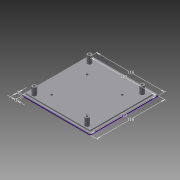
# Autodesk Inventor part: nuccase_top
Saved by Autodesk Inventor 2015 (Build 190159000, 159)
## iProperties
Created: 2016-10-24
Part Number: nuccase_top
Material: Generic
Document SubType Name: Modeling
Designer: Bardo91
Density: 1 g/cm^3
Appearance: Default
Author: Bardo91
Autodesk Inventor part; units mm, degrees
ref_plane "YZ Plane" through (0, 0, 0) normal (1, 0, 0) x (0, 1, 0)
ref_plane "XZ Plane" through (0, 0, 0) normal (0, 1, 0) x (-1, 0, 0)
ref_plane "XY Plane" through (0, 0, 0) normal (0, 0, 1) x (1, 0, 0)
sketch "Sketch1" plane through (0, 0, 0) normal (0, 0, 1) x (1, 0, 0)
  line L0 (0, 0) -> (110, 0)
  line L1 (110, 0) -> (110, 110)
  line L2 (110, 110) -> (0, 110)
  line L3 (0, 110) -> (0, 0)
  line L4 (0, 0) -> (0, -3)
  line L5 (0, -3) -> (-3, -3)
  line L6 (-3, -3) -> (113, -3)
  line L7 (113, -3) -> (113, 113)
  line L8 (113, 113) -> (-3, 113)
  line L9 (-3, 113) -> (-3, -3)
  dimension "d0" = 110
  dimension "d1" = 110
  dimension "d2" = 3
  dimension "d3" = 3
  dimension "d4" = 116
  dimension "d5" = 116
  constraints: 20 end point, 4 parallel, 3 perpendicular, 2 horizontal, 1 vertical
  measures "d0" distance of L2.end L1.end
  measures "d1" distance of L1.end L0.end
  measures "d2" distance of L0.start L4.end
  measures "d3" distance of L4.end L5.end
  measures "d4" distance of L8.end L7.end
  measures "d5" distance of L7.end L6.end
extrude "Extrusion1" add sketch "Sketch1" along normal blind 4 contours L3 L2 L1 L0
extrude "Extrusion2" add sketch "Sketch1" along normal blind 2
sketch "Sketch2" plane through (0, 0, 4) normal (0, 0, 1) x (1, 0, 0)
  line L0 (0, 0) -> (110, 0) projected
  line L1 (55, 0) -> (55, 5)
  line L2 (55, 5) -> (10, 5)
  line L3 (10, 5) -> (100, 5)
  line L4 (100, 5) -> (100, 99)
  line L5 (100, 99) -> (10, 99)
  circle A0 centre (10, 99) radius 3.5
  circle A1 centre (100, 99) radius 3.5
  circle A2 centre (100, 5) radius 3.5
  circle A3 centre (10, 5) radius 3.5
  dimension "d10" = 5
  dimension "d11" = 45
  dimension "d12" = 90
  dimension "d13" = 94
  dimension "d14" = 90
  dimension "d15" = 7
  dimension "d16" = 7
  dimension "d17" = 7
  dimension "d18" = 7
  constraints: 10 end point, 4 centre point, 4 coincident, 3 perpendicular, 1 midpoint, 1 point on line, 1 vertical
  measures "d10" distance of L1.start L1.end
  measures "d11" distance of L1.end L2.end
  measures "d12" distance of L2.end L3.end
  measures "d13" distance of L3.end L4.end
  measures "d14" distance of L4.end L5.end
  measures "d15" diameter of A0
  measures "d16" diameter of A1
  measures "d17" diameter of A2
  measures "d18" diameter of A3
extrude "Extrusion3" add sketch "Sketch2" along normal blind 13
sketch "Sketch3" plane through (10, 99, 17) normal (0, 0, 1) x (1, 0, 0)
  circle A0 centre (0, -94) radius 3.5 projected
  circle A1 centre (0, -94) radius 1.75
  circle A2 centre (90, -94) radius 3.5 projected
  circle A3 centre (90, -94) radius 1.75
  circle A4 centre (90, 0) radius 3.5 projected
  circle A5 centre (90, 0) radius 1.75
  circle A6 centre (0, 0) radius 1.75
  point P0 (-10, -99)
  dimension "d21" = 3.5
  dimension "d22" = 3.5
  dimension "d23" = 3.5
  dimension "d24" = 3.5
  constraints: 4 centre point, 3 coincident
  measures "d21" diameter of A1
  measures "d22" diameter of A3
  measures "d23" diameter of A5
  measures "d24" diameter of A6
extrude "Extrusion4" cut sketch "Sketch3" against normal through all contours A1 | A3 | A5 | A6
sketch "Sketch4" plane through (0, 0, 4) normal (0, 0, 1) x (1, 0, 0)
  line L0 (0, 0) -> (110, 0) projected
  line L1 (55, 0) -> (55, 20)
  line L2 (55, 20) -> (85, 20)
  line L3 (85, 20) -> (85, 80)
  line L4 (85, 80) -> (25, 80)
  line L5 (25, 80) -> (25, 20)
  circle A0 centre (25, 80) radius 1.75
  circle A1 centre (85, 80) radius 1.75
  circle A2 centre (85, 20) radius 1.75
  circle A3 centre (25, 20) radius 1.75
  dimension "d27" = 20
  dimension "d28" = 30
  dimension "d29" = 60
  dimension "d30" = 60
  dimension "d31" = 60
  dimension "d32" = 3.5
  dimension "d33" = 3.5
  dimension "d34" = 3.5
  dimension "d35" = 3.5
  constraints: 10 end point, 4 centre point, 4 coincident, 3 perpendicular, 1 midpoint, 1 point on line, 1 vertical
  measures "d27" distance of L1.start L1.end
  measures "d28" distance of L1.end L2.end
  measures "d29" distance of L2.end L3.end
  measures "d30" distance of L3.end L4.end
  measures "d31" distance of L4.end L5.end
  measures "d32" diameter of A0
  measures "d33" diameter of A1
  measures "d34" diameter of A2
  measures "d35" diameter of A3
extrude "Extrusion5" cut sketch "Sketch4" against normal blind 15
body "Solid1"
